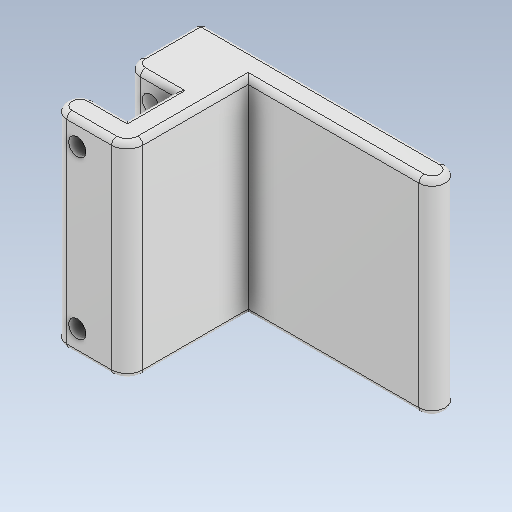
# Autodesk Inventor part: ハンド3D_L
Saved by Autodesk Inventor 2020.3 (Build 243373000, 373)
## iProperties
Created: 2020-07-06
Part Number: ハンド3D_L
Material: ABS プラスチック
Document SubType Name: Modeling
Designer: totot
Mass: 18.9718 g
Surface Area: 77.0508 cm^2
Volume: 17.8979 cm^3
Density: 1.06 g/cm^3
Appearance: 滑らか - 白
Author: totot
Autodesk Inventor part; units mm, degrees
ref_plane "YZ Plane" through (0, 0, 0) normal (1, 0, 0) x (0, 1, 0)
ref_plane "XZ Plane" through (0, 0, 0) normal (0, 1, 0) x (-1, 0, 0)
ref_plane "XY Plane" through (0, 0, 0) normal (0, 0, 1) x (1, 0, 0)
sketch "スケッチ1" plane through (0, 0, 0) normal (0, 0, 1) x (1, 0, 0)
  line L0 (0, 0) -> (49, 0)
  line L1 (49, 0) -> (49, -39)
  line L2 (49, -39) -> (0, -39)
  line L3 (0, -39) -> (0, 0)
  dimension "d2" = 39
  dimension "d3" = 49
  constraints: 8 end point, 2 parallel, 1 horizontal, 1 perpendicular
  measures "d2" distance of L2.end L0.start
  measures "d3" distance between parallel lines of L3 L1
extrude "押し出し1" add sketch "スケッチ1" along normal blind 5
sketch "スケッチ2" plane through (0, 0, 5) normal (0, 0, 1) x (1, 0, 0)
  line L0 (49, 0) -> (0, 0) projected
  line L1 (9, 0) -> (14, 0)
  line L2 (14, 0) -> (14, -39)
  line L3 (14, -39) -> (9, -39)
  line L4 (9, -39) -> (9, 0)
  line L5 (0, 0) -> (0, -39) projected
  dimension "d4" = 5
  dimension "d5" = 39
  dimension "d6" = 9
  constraints: 8 end point, 2 parallel, 1 horizontal, 1 perpendicular, 1 point on line
  measures "d4" distance of L2.end L3.end
  measures "d5" distance of L1.end L2.end
  measures "d6" distance between parallel lines of L4 L5
extrude "押し出し2" add sketch "スケッチ2" along normal blind 9
sketch "スケッチ3" plane through (0, 0, 14) normal (0, 0, 1) x (1, 0, 0)
  line L0 (0, -39) -> (9, -39) projected
  line L1 (14, 0) -> (0, 0)
  line L2 (0, 0) -> (0, -39)
  line L3 (0, -39) -> (14, -39)
  line L4 (14, -39) -> (14, 0)
  point P0 (0, 0)
  constraints: 8 end point, 2 parallel, 1 horizontal, 1 perpendicular
extrude "押し出し3" add sketch "スケッチ3" along normal blind 5
sketch "スケッチ4" plane through (0, 0, 0) normal (0, 0, -1) x (-1, 0, 0)
  line L0 (-49, 0) -> (-14, 0) projected
  line L1 (0, -39) -> (-49, -39) projected
  line L2 (-49, 0) -> (0, 0)
  line L3 (0, 0) -> (0, -39)
  line L4 (0, -39) -> (-49, -39)
  line L5 (-49, -39) -> (-49, 0)
  point P0 (0, 0)
  constraints: 8 end point, 2 parallel, 1 horizontal, 1 perpendicular
extrude "押し出し4" add sketch "スケッチ4" along normal blind 9
sketch "スケッチ5" plane through (0, 0, 5) normal (0, 0, 1) x (1, 0, 0)
  line L0 (49, 0) -> (14, 0) projected
  line L1 (14, 0) -> (49, 0)
  line L2 (49, 0) -> (49, -39)
  line L3 (49, -39) -> (14, -39)
  line L4 (14, -39) -> (14, 0)
  point P0 (0, 0)
  constraints: 8 end point, 2 parallel, 1 horizontal, 1 perpendicular
extrude "押し出し5" cut sketch "スケッチ5" against normal blind 9
fillet "フィレット1" radius 2.5 2 edges at (49, -19.5, -4) (49, -19.5, -9)
fillet "フィレット2" radius 2.5 3 edges at (0, -19.5, 19) (0, -19.5, 14) (0, -19.5, 5)
sketch "スケッチ6" plane through (0, 0, -9) normal (0, 0, -1) x (-1, 0, 0)
  line L0 (0, 0) -> (-46.5, 0) projected
  line L1 (-46.5, -39) -> (0, -39) projected
  line L2 (0, -39) -> (0, 0) projected
  point P0 (-4.5, -4.5)
  point P1 (-4.5, -34.5)
  dimension "d17" = 4.5
  dimension "d18" = 4.5
  dimension "d19" = 4.5
  dimension "d20" = 4.5
  measures "d17" distance from line of point (-4.5, -4.5) L0
  measures "d18" distance from line of L1 point (-4.5, -34.5)
  measures "d19" distance from line of point (-4.5, -34.5) L2
  measures "d20" distance from line of point (-4.5, -4.5) L2
hole "穴1" at (4.5, -4.5, -9) at (4.5, -34.5, -9) direction (0, 0, 1) diameter 3.3 end through all counterbore diameter 6 counterbore depth 8
fillet "フィレット5" radius 1 23 edges at (48.2678, 0, -4.7322) (30.2501, 0, -4) (23.25, 0, -9) (0.7322, 0, 4.2678) (5.7499, 0, 5) (0, 0, -3.2499) (9, 0, 9.5) (14, 0, 7.5) (0.7322, 0, 18.2678) (5.75, 0, 14) (8.25, 0, 19) (0, -19.5, -9) (48.2678, -39, -4.7322) (30.2501, -39, -4) (23.2501, -39, -9) (9, -39, 9.5) (0.7322, -39, 18.2678) (8.25, -39, 19) (5.75, -39, 14) (5.75, -39, 5) (0, -39, -3.25) (0.7322, -39, 4.2678) (14, -39, 7.5)
fillet "フィレット6" radius 3 3 edges at (13.7071, -0.2929, 18.7071) (13.7071, -38.7071, 18.7071) (14, -19.5, 19)
equation "\"d18\" = d17"
equation "\"d19\" = d18"
equation "\"d20\" = d17"
